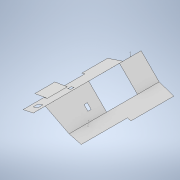
# Autodesk Inventor part: mainPartHouseRoofV2
Saved by Autodesk Inventor 2022.1 (Build 261234000, 234)
## iProperties
Created: 2021-07-13
Part Number: mainPartHouseRoofV2
Material: Generic
Document SubType Name: Modeling
Designer: robst
Density: 1 g/cm^3
Appearance: Default
Author: robst
Autodesk Inventor part; units mm, degrees
ref_plane "Work Plane3" through (0, 0, 0) normal (-0.7071068, 0.7071068, 0) x (0, 0, 1)
sketch "Sketch8" plane through (0, 0, 0) normal (-0.7071068, 0.7071068, 0) x (0, 0, 1)
  line L0 (0, 0) -> (-17526, 0)
  line L1 (-17526, 0) -> (-17526, -4699)
  line L2 (-17526, -4699) -> (-13538.2, -4699)
  line L3 (-13538.2, -4699) -> (-13538.2, 0)
  line L4 (-7874, 0) -> (-7874, -4699)
  line L5 (-7874, -4699) -> (-1127.76, -4699)
  line L6 (-1127.76, -4699) -> (0, 0)
  line L7 (0, 0) -> (0, -3810) construction
  point P0 (-13538.2, -2349.5)
  dimension "d39" = 17526
  dimension "d40" = 4699
  dimension "d41" = 3987.8
  dimension "d42" = 5664.2
  constraints: 16 end point, 3 vertical, 2 horizontal, 2 perpendicular, 2 point on line, 1 collinear, 1 midpoint
  measures "d39" distance of L0.start L0.end
  measures "d40" distance of L0.end L1.end
  measures "d41" distance of L1.end L2.end
  measures "d42" distance from line of L4 point (-13538.2, -2349.5)
ref_plane "Work Plane5" through (-3322.6948, -3322.6948, -17526) normal (-0.3162278, 0.9486833, 0) x (0, 0, 1)
sketch "Sketch9" plane through (-3322.6948, -3322.6948, -17526) normal (-0.3162278, 0.9486833, 0) x (0, 0, 1)
  line L0 (1.5493, 7.5954) -> (16613.8771, 7.5954)
  line L1 (1.5493, 7.5954) -> (1.5493, -2964.2046)
  line L2 (1.5493, -2964.2046) -> (4751.3493, -2964.2046)
  line L3 (4751.3493, -2964.2046) -> (4751.3493, -2329.2046)
  line L4 (4751.3493, -2329.2046) -> (8610.6611, -2329.2046)
  line L5 (8610.6611, -2329.2046) -> (8610.6611, -1643.4046)
  line L6 (8610.6611, -1643.4046) -> (12268.2611, -1643.4046)
  line L7 (12268.2611, -1643.4046) -> (12268.2611, -2329.2046)
  line L8 (12268.2611, -2329.2046) -> (16052.8611, -2329.2046)
  line L9 (9042.4611, -1110.0046) -> (9042.4611, -500.4046)
  line L10 (9042.4611, -500.4046) -> (8432.8611, -500.4046)
  line L11 (8432.8611, -500.4046) -> (8432.8611, -1110.0046)
  line L12 (8432.8611, -1110.0046) -> (9042.4611, -1110.0046)
  line L13 (9042.4611, -1110.0046) -> (8432.8611, -500.4046) construction
  line L14 (9042.4611, -500.4046) -> (8432.8611, -1110.0046) construction
  line L15 (14051.3887, -1541.8046) -> (14953.0887, -1541.8046)
  line L16 (14051.3887, -1541.8046) -> (14041.1454, -627.462)
  line L17 (14041.1454, -627.462) -> (14936.1378, -602.1575)
  line L18 (14936.1378, -602.1575) -> (14953.0887, -1541.8046)
  line L19 (-3503.3408, 4202.9134) -> (21030.8901, 4202.9134) projected
  line L20 (14488.6416, -614.8098) -> (14488.6416, 7.5954)
  line L21 (17526, 4202.9134) -> (17526, -2329.2046) construction
  line L22 (16052.8611, -2329.2046) -> (16405.5971, 7.5954)
  point P0 (8737.6611, -805.2046)
  point P1 (8737.6611, -500.4046)
  point P2 (14049.7848, -2336.9504)
  point P3 (14647.0941, -2336.9504)
  dimension "d50" = 2971.8
  dimension "d51" = 4749.8
  dimension "d52" = 635
  dimension "d59" = 16612.3278
  dimension "d60" = 3784.6
  dimension "d61" = 3657.6
  dimension "d81" = 609.6
  dimension "d84" = 901.7
  dimension "d85" = 914.4
  dimension "d86" = 939.8
  dimension "d87" = 895.35
  dimension "d90" = 4195.318
  dimension "d103" = 431.8
  dimension "d104" = 787.4
  dimension "d105" = 787.4
  dimension "d106" = 1651
  dimension "d111" = 1219.2
  dimension "d112" = 912.1229
  dimension "d115" = 208.28
  constraints: 44 end point, 9 perpendicular, 4 midpoint, 4 point on line, 3 parallel, 2 horizontal, 2 vertical
  measures "d50" distance of L0.start L1.end
  measures "d51" distance of L1.end L2.end
  measures "d52" distance of L2.end L3.end
  measures "d59" distance of L0.end L0.start
  measures "d60" distance of L7.end L8.end
  measures "d61" distance of L5.end L6.end
  measures "d81" distance of L9.end L10.end
  measures "d84" distance of L15.start L15.end
  measures "d85" distance of L15.start L16.end
  measures "d86" distance of L17.end L15.end
  measures "d87" distance of L16.end L17.end
  measures "d90" distance between parallel lines of L0 L19
  measures "d103" distance from line of L9.start L5
  measures "d104" distance from line of L15.start L8
  measures "d105" distance from line of L15.end L8
  measures "d106" distance between parallel lines of L6 L0
  measures "d111" distance between parallel lines of L12 L4
  measures "d112" distance from line of L0.end L21
  measures "d115" distance of L22.end L0.end
ref_plane "Work Plane6" through (0, 0, 0) normal (0.7071068, 0.7071068, 0) x (0, 0, 1)
sketch "Sketch11" plane through (0, 0, 0) normal (0.7071068, 0.7071068, 0) x (0, 0, 1)
  line L0 (0, 0) -> (-17526, 0)
  line L1 (-17526, 0) -> (-17526, 4648.2)
  line L2 (0, 0) -> (-1066.8, 4648.2)
  line L3 (-13563.6, 0) -> (-13563.6, 4648.2)
  line L4 (-7924.8, 0) -> (-7924.8, 4648.2)
  line L5 (-17526, 4648.2) -> (-13563.6, 4648.2)
  line L6 (-7924.8, 4648.2) -> (-1066.8, 4648.2)
  line L7 (-5435.6, 3340.1) -> (-6019.8, 3340.1)
  line L8 (-6019.8, 3340.1) -> (-6019.8, 2324.1)
  line L9 (-6019.8, 2324.1) -> (-5435.6, 2324.1)
  line L10 (-5435.6, 2324.1) -> (-5435.6, 3340.1)
  line L11 (-5435.6, 3340.1) -> (-6019.8, 2324.1) construction
  line L12 (-6019.8, 3340.1) -> (-5435.6, 2324.1) construction
  point P0 (-5727.7, 2832.1)
  point P1 (-6019.8, 2832.1)
  dimension "d63" = 17526
  dimension "d65" = 4648.2
  dimension "d66" = 16459.2
  dimension "d67" = 77.074
  dimension "d74" = 3962.4
  dimension "d75" = 5638.8
  dimension "d116" = 584.2
  dimension "d117" = 1016
  dimension "d118" = 1905
  constraints: 26 end point, 7 perpendicular, 3 midpoint, 2 horizontal, 2 parallel, 2 point on line, 1 vertical
  measures "d63" distance of L0.start L0.end
  measures "d65" distance of L0.end L1.end
  measures "d66" distance of L1.end L2.end
  measures "d67" angle of L2 L0
  measures "d74" distance between parallel lines of L3 L1
  measures "d75" distance between parallel lines of L4 L3
  measures "d116" distance of L8.end L9.end
  measures "d117" distance of L9.end L7.start
  measures "d118" distance from line of point (-6019.8, 2832.1) L4
ref_plane "Work Plane8" through (3286.7737, -3286.7737, -17526) normal (0.3162278, 0.9486833, 0) x (0, 0, 1)
sketch "Sketch13" plane through (3286.7737, -3286.7737, -17526) normal (0.3162278, 0.9486833, 0) x (0, 0, 1)
  line L0 (0, 0) -> (16459.206, 0)
  line L1 (0, 0) -> (0, 2844.8)
  line L2 (0, 2844.8) -> (7874, 2844.8)
  line L3 (7874, 2844.8) -> (7874, 2209.8)
  line L4 (7874, 2209.8) -> (16332.2, 2209.8)
  line L5 (16332.2, 2209.8) -> (16459.206, 0)
  point P0 (17526, -4157.4765)
  dimension "d77" = 2844.8
  dimension "d78" = 7874
  dimension "d79" = 635
  dimension "d80" = 8458.2
  dimension "d127" = 2209.8
  constraints: 12 end point, 3 perpendicular, 1 horizontal, 1 vertical
  measures "d77" distance of L0.start L1.end
  measures "d78" distance of L1.end L2.end
  measures "d79" distance of L2.end L3.end
  measures "d80" distance of L3.end L4.end
  measures "d127" distance between parallel lines of L4 L0
extrude "Extrusion12" add sketch "Sketch9" against normal blind 0.0254
extrude "Extrusion13" add sketch "Sketch8" against normal blind 0.0254
extrude "Extrusion15" add sketch "Sketch13" against normal blind 0.0254
ref_plane "Work Plane9" through (-4881.7653, -3842.3849, -8915.3389) normal (-0.164399, 0.9863939, 0) x (0, 0, 1)
sketch "Sketch14" plane through (-4881.7653, -3842.3849, -8915.3389) normal (-0.164399, 0.9863939, 0) x (0, 0, 1)
  line L0 (3657.6, -677.4039) -> (3657.6, 0.004) projected
  line L1 (3657.6, 0.004) -> (0, 0.004) projected
  line L2 (3657.6, 0.004) -> (0, 0.004)
  line L3 (0, 0.004) -> (0, -2311.396)
  line L4 (0, -2311.396) -> (3657.6, -2311.396)
  line L5 (3657.6, -2311.396) -> (3657.6, 0.004)
  point P0 (8915.3389, 5447.0278)
  point P1 (1828.8, -2311.396)
  dimension "d108" = 2311.4
  constraints: 8 end point, 3 perpendicular, 1 collinear, 1 midpoint
  measures "d108" distance from line of point (1828.8, -2311.396) L1
extrude "Extrusion16" add sketch "Sketch14" against normal blind 0.0254
extrude "Extrusion17" add sketch "Sketch11" against normal blind 0.0254
ref_plane "Work Plane10" through (-6573.5475, 0, 0) normal (0.1601822, 0.9870875, 0) x (0, 0, -1)
sketch "Sketch15" plane through (-6573.5475, 0, 0) normal (0.1601822, 0.9870875, 0) x (0, 0, -1)
  circle A0 centre (3439.4375, -11218.9268) radius 25.4
  point P0 (0, -6488.6663)
  dimension "d121" = 50.8
  constraints: 1 centre point
  measures "d121" diameter of A0
extrude "Extrusion18" add sketch "Sketch15" against normal blind 914.4
sketch "Sketch16" plane through (0, 0, 0) normal (0, 1, 0) x (-1, 0, 0)
  circle A0 centre (799.9669, -16299.3246) radius 25.4
  point P0 (0, 0)
  dimension "d124" = 50.8
  constraints: 1 centre point
  measures "d124" diameter of A0
extrude "Extrusion19" add sketch "Sketch16" against normal blind 914.4
equation "\"d39\" = mainRidgeLine"
equation "\"d40\" = ridgeLineToGarargeEaveAtBackOfHouse"
equation "\"d41\" = backOfHouseToBackOfDormer"
equation "\"d42\" = dormerLengthOnGarageSide"
equation "\"d52\" = garageSideCantalever"
equation "\"d61\" = porchLength"
equation "\"d63\" = mainRidgeLine"
equation "\"d66\" = lengthBackOfHouseToFrontPoolSideAlongTransition"
equation "\"d78\" = lengthBackOfHouseToCantaleverPoolSide"
equation "\"d79\" = poolSideCanterlever"
equation "\"d91\" = extrusionForDrawing"
equation "\"d93\" = extrusionForDrawing"
equation "\"d97\" = extrusionForDrawing"
equation "\"d109\" = extrusionForDrawing"
equation "\"d119\" = extrusionForDrawing"
equation "\"pitch_4_12\" = 18.434949deg"
equation "\"pitch_12_12\" = 45deg"
equation "\"pitch_2_12\" = 9.462322deg"
equation "\"d38\" = pitch_12_12"
equation "\"mainRidgeLine\" = 17526"
equation "\"ridgeLineToGarargeEaveAtBackOfHouse\" = 4699"
equation "\"backOfHouseToBackOfDormer\" = 3987.8"
equation "\"dormerLengthOnGarageSide\" = 5664.2"
equation "\"lengthGarageEveToTransitionAtBackOfHouse\" = 2971.8"
equation "\"d62\" = -pitch_12_12"
equation "\"garageSideCantalever\" = 635"
equation "\"poolSideCanterlever\" = 635"
equation "\"porchLength\" = 3657.6"
equation "\"lengthBackOfHouseToFrontPoolSideAlongTransition\" = 16459.2"
equation "\"lengthBackOfHouseToCantaleverPoolSide\" = 7874"
equation "\"lenghtCantaleverToFrontPoolSide\" = 7366"
equation "\"d76\" = -pitch_4_12"
equation "\"extrusionForDrawing\" = 0.0254"
equation "\"d107\" = pitch_2_12"
body "Solid5"
